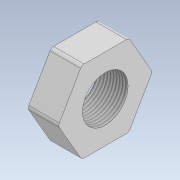
# Autodesk Inventor part: tuerca
Saved by Autodesk Inventor 2021 (Build 250183000, 183)
## iProperties
Created: 2021-04-24
Part Number: tuerca
Material: Genérico
Document SubType Name: Modeling
Designer: j2seb
Density: 1 g/cm^3
Appearance: Valor por defecto
Author: j2seb
Autodesk Inventor part; units mm, degrees
ref_plane "YZ Plane" through (0, 0, 0) normal (1, 0, 0) x (0, 1, 0)
ref_plane "XZ Plane" through (0, 0, 0) normal (0, 1, 0) x (-1, 0, 0)
ref_plane "XY Plane" through (0, 0, 0) normal (0, 0, 1) x (1, 0, 0)
sketch "Boceto1" plane through (0, 0, 0) normal (1, 0, 0) x (0, 1, 0)
  line L0 (20, 11.547) -> (20, -11.547)
  line L1 (20, 11.547) -> (0, 0) construction
  line L2 (0, 0) -> (20, -11.547) construction
  line L3 (0, 0) -> (20, 11.547) construction
  line L4 (0, 23.094) -> (20, 11.547)
  line L5 (0, 23.094) -> (0, 0) construction
  line L6 (0, 0) -> (0, 23.094) construction
  line L7 (-20, 11.547) -> (0, 23.094)
  line L8 (-20, 11.547) -> (0, 0) construction
  line L9 (0, 0) -> (-20, 11.547) construction
  line L10 (-20, -11.547) -> (-20, 11.547)
  line L11 (-20, -11.547) -> (0, 0) construction
  line L12 (0, 0) -> (-20, -11.547) construction
  line L13 (0, -23.094) -> (-20, -11.547)
  line L14 (0, -23.094) -> (0, 0) construction
  line L15 (0, 0) -> (0, -23.094) construction
  line L16 (20, -11.547) -> (0, -23.094)
  line L17 (20, -11.547) -> (0, 0) construction
  point P0 (20, 0)
  point P1 (10, 17.3205)
  point P2 (-10, 17.3205)
  point P3 (-20, 0)
  point P4 (-10, -17.3205)
  point P5 (10, -17.3205)
  point P6 (20, 11.547)
  point P7 (0, 23.094)
  point P8 (-20, 11.547)
  point P9 (-20, -11.547)
  point P10 (0, -23.094)
  point P11 (20, -11.547)
  dimension "d1" = 60
  dimension "d2" = 20
  dimension "d5" = 360
  constraints: 36 end point, 3 coincident, 1 horizontal alignment, 1 midpoint, 1 vertical, 41 other
  measures "d1" angle of L2 L1
  measures "d2" distance from line of L1.end L0
extrude "Extrusión1" add sketch "Boceto1" along normal blind 15
hole "Agujero1" at (0, 0, 0) direction (1, 0, 0) diameter 22.3762 end through all thread size "M24x1.5" class "6H" standard "ISO Metric profile"
fillet "Empalme1" radius 2 6 edges at (7.5, 20, -11.547) (7.5, 0, -23.094) (7.5, -20, -11.547) (7.5, 20, 11.547) (7.5, 0, 23.094) (7.5, -20, 11.547)
